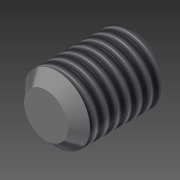
# Autodesk Inventor part: SetScrew3
Saved by Autodesk Inventor 2015 (Build 190159000, 159)
## iProperties
Created: 2014-07-10
Part Number: SetScrew3
Material: Steel, Alloy
Document SubType Name: Modeling
Designer: t_clevj
Density: 7.73 g/cm^3
Appearance: Semi-Polished
Author: t_clevj
Autodesk Inventor part; units mm, degrees
ref_plane "YZ Plane" through (0, 0, 0) normal (1, 0, 0) x (0, 1, 0)
ref_plane "XZ Plane" through (0, 0, 0) normal (0, 1, 0) x (-1, 0, 0)
ref_plane "XY Plane" through (0, 0, 0) normal (0, 0, 1) x (1, 0, 0)
sketch "Sketch1" plane through (0, 0, 0) normal (0, 1, 0) x (-1, 0, 0)
  circle A0 centre (0, 0) radius 1.5
  dimension "d0" = 3
  constraints: 1 centre point, 1 coincident
  measures "d0" diameter of A0
extrude "Extrusion1" add sketch "Sketch1" along normal blind 4
sketch "Sketch2" plane through (0, 4, 0) normal (0, 1, 0) x (1, 0, 0)
  circle A0 centre (0, 0) radius 1.5 projected
  line L0 (0.75, -0.433) -> (0, -0.866)
  line L1 (0, -0.866) -> (-0.75, -0.433)
  line L2 (-0.75, -0.433) -> (-0.75, 0.433)
  line L3 (-0.75, 0.433) -> (0, 0.866)
  line L4 (0, 0.866) -> (0.75, 0.433)
  line L5 (0.75, 0.433) -> (0.75, -0.433)
  dimension "d3" = 1.5
  constraints: 12 end point, 1 coincident, 1 vertical, 13 other
  measures "d3" distance between parallel lines of L2 L5
extrude "Extrusion2" cut sketch "Sketch2" against normal blind 1.2 contours L0 L1 L2 L3 L4 L5
chamfer "Chamfer1" distance 0.5 angle 45 1 edges at (1.5, 0, 0)
thread "Thread1" size "M3x0.5" class "6g" standard "ANSI Metric M Profile" full length
chamfer "Chamfer2" distance 0.2 angle 45 7 edges at (1.5, 4, 0) (-0.75, 4, 0) (-0.375, 4, -0.6495) (0.375, 4, -0.6495) (0.75, 4, 0) (0.375, 4, 0.6495) (-0.375, 4, 0.6495)
body "Solid1"
